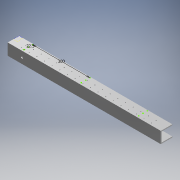
# Autodesk Inventor part: X-portal-front-plate
Saved by Autodesk Inventor 2016 (Build 200138000, 138)
## iProperties
Created: 2015-04-18
Part Number: X-portal-front-plate
Material: Aluminum 6061
Document SubType Name: Modeling
Designer: shu
Density: 2.7 g/cm^3
Appearance: Aluminum - Flat
Mass: 1937.89 g
Surface Area: 2815.57 cm^2
Volume: 717.738 cm^3
Author: shu
Autodesk Inventor part; units mm, degrees
ref_plane "YZ Plane" through (0, 0, 0) normal (1, 0, 0) x (0, 1, 0)
ref_plane "XZ Plane" through (0, 0, 0) normal (0, 1, 0) x (-1, 0, 0)
ref_plane "XY Plane" through (0, 0, 0) normal (0, 0, 1) x (1, 0, 0)
sketch "Sketch1" plane through (0, 0, 0) normal (0, 0, 1) x (1, 0, 0)
  line L0 (0, 0) -> (800, 0)
  line L1 (800, 0) -> (800, -60)
  line L2 (800, -60) -> (0, -60)
  line L3 (0, -60) -> (0, 0)
  dimension "d0" = 800
  dimension "d1" = 60
  constraints: 8 end point, 2 parallel, 1 horizontal, 1 perpendicular
  measures "d0" distance of L1.end L2.end
  measures "d1" distance of L0.end L1.end
extrude "Extrusion1" add sketch "Sketch1" along normal blind 5
sketch "Sketch13" plane through (0, 0, 0) normal (0, 0, -1) x (-1, 0, 0)
  line L0 (0, -60) -> (-800, -60) projected
  line L1 (0, -60) -> (-800, -60)
  line L2 (-800, -60) -> (-800, -55)
  line L3 (-800, -55) -> (0, -55)
  line L4 (0, -55) -> (0, -60)
  point P0 (0, 0)
  dimension "d65" = 800
  dimension "d66" = 5
  constraints: 8 end point, 2 parallel, 1 horizontal, 1 perpendicular
  measures "d65" distance of L2.end L3.end
  measures "d66" distance of L1.end L2.end
extrude "Extrusion12" add sketch "Sketch13" along normal blind 55
sketch "Sketch14" plane through (0, 0, 5) normal (0, 0, 1) x (1, 0, 0)
  line L0 (60, 0) -> (60, -60) construction
  line L1 (0, -60) -> (800, -60) construction
  line L2 (0, -55) -> (0, 0) construction
  point P0 (60, -48)
  point P1 (60, -25)
  dimension "d71" = 60
  constraints: 3 point on line, 2 end point, 1 vertical
  measures "d71" distance from line of L2 point (60, -25)
hole "Hole1" at (60, -48, 5) at (60, -25, 5) direction (0, 0, -1) diameter 4 end through all
pattern_linear "Rectangular Pattern1" count 18 spacing 40 along (1, 0, 0) of "Hole1"
sketch "Sketch15" plane through (0.5, -55, -55) normal (0, 1, 0) x (1, 0, 0)
  line L0 (799.5, 0) -> (-0.5, 0) projected
  line L1 (-0.5, 0) -> (799.5, 0)
  line L2 (799.5, 0) -> (799.5, -5)
  line L3 (799.5, -5) -> (-0.5, -5)
  line L4 (-0.5, -5) -> (-0.5, 0)
  point P0 (-0.5, -55)
  dimension "d91" = 800
  dimension "d92" = 5
  constraints: 8 end point, 2 parallel, 1 horizontal, 1 perpendicular
  measures "d91" distance of L2.end L3.end
  measures "d92" distance of L1.end L2.end
extrude "Extrusion13" add sketch "Sketch15" along normal up to surface (55 mm away)
sketch "Sketch19" plane through (0, -60, 5) normal (0, -1, 0) x (1, 0, 0)
  point P0 (75, -30)
hole "Hole7" at (75, -60, -25) direction (0, 1, 0) diameter 5.3 depth 5 counterbore diameter 10 counterbore depth 3.5
sketch "Sketch20" plane through (0, 0, 5) normal (0, 0, 1) x (1, 0, 0)
  line L0 (0, 0) -> (21.0571, 0) construction
  line L1 (21.0571, 0) -> (21.0571, -30.3151) construction
  line L2 (21.0571, -30.3151) -> (0, -30.3151) construction
  line L3 (0, -30.3151) -> (0, 0) construction
  point P0 (75, -5)
  point P1 (375, -5)
  point P2 (675, -5)
  point P3 (75, -27.5)
  point P4 (375, -27.5)
  point P5 (675, -27.5)
  point P6 (75, -50)
  point P7 (375, -50)
  point P8 (675, -50)
  dimension "d123" = 300
  dimension "d126" = 22.5
  constraints: 8 end point, 2 horizontal, 2 parallel, 1 perpendicular, 1 vertical, 8 other
  measures "d123" distance of point (75, -5) point (375, -5)
  measures "d126" distance of point (75, -5) point (75, -27.5)
sketch "Sketch21" plane through (0, 0, 5) normal (0, 0, 1) x (1, 0, 0)
  point P0 (75, -50)
  point P1 (375, -27.5)
  point P2 (375, -50)
  point P3 (375, -5)
  point P4 (675, -5)
  point P5 (675, -27.5)
  point P6 (675, -50)
  point P7 (75, -5)
  point P8 (75, -27.5)
hole "Hole9" at (75, -50, 5) at (375, -27.5, 5) at (375, -50, 5) at (375, -5, 5) at (675, -5, 5) at (675, -27.5, 5) at (675, -50, 5) at (75, -5, 5) at (75, -27.5, 5) direction (0, 0, -1) diameter 5.5 depth 5
sketch "Sketch22" plane through (0, 0, -55) normal (0, 0, -1) x (-1, 0, 0)
  line L0 (0, 0) -> (-32.4648, 0) construction
  line L1 (-32.4648, 0) -> (-32.4648, -15.4297) construction
  line L2 (-32.4648, -15.4297) -> (0, -15.4297) construction
  line L3 (0, -15.4297) -> (0, 0) construction
  point P0 (-75, -5)
  point P1 (-375, -5)
  point P2 (-675, -5)
  point P3 (-75, -27.5)
  point P4 (-375, -27.5)
  point P5 (-675, -27.5)
  point P6 (-75, -50)
  point P7 (-375, -50)
  point P8 (-675, -50)
  dimension "d138" = 300
  dimension "d141" = 22.5
  constraints: 8 end point, 2 horizontal, 2 parallel, 1 perpendicular, 1 vertical, 8 other
  measures "d138" distance of point (-75, -5) point (-375, -5)
  measures "d141" distance of point (-75, -5) point (-75, -27.5)
hole "Hole11" at (75, -27.5, -55) at (75, -5, -55) at (75, -50, -55) at (375, -50, -55) at (375, -27.5, -55) at (375, -5, -55) at (675, -27.5, -55) at (675, -5, -55) at (675, -50, -55) direction (0, 0, 1) diameter 5 depth 5 tip angle 118
sketch "Sketch23" plane through (0, 0, 0) normal (0, 1, 0) x (1, 0, 0)
  point P0 (200, 52.5)
  point P1 (200, -2.5)
  point P2 (250, -2.5)
  point P3 (300, 52.5)
  point P4 (300, -2.5)
  point P5 (350, 52.5)
  point P6 (350, -2.5)
  point P7 (400, 52.5)
  point P8 (400, -2.5)
  point P9 (450, 52.5)
  point P10 (450, -2.5)
  point P11 (500, 52.5)
  point P12 (500, -2.5)
  point P13 (550, 52.5)
  point P14 (550, -2.5)
  point P15 (600, 52.5)
  point P16 (600, -2.5)
  point P17 (650, 52.5)
  point P18 (650, -2.5)
  point P19 (250, 52.5)
  point P20 (100, 52.5)
  point P21 (100, -2.5)
  point P22 (150, 52.5)
  point P23 (150, -2.5)
hole "Hole12" at (200, 0, -52.5) at (200, 0, 2.5) at (250, 0, 2.5) at (300, 0, -52.5) at (300, 0, 2.5) at (350, 0, -52.5) at (350, 0, 2.5) at (400, 0, -52.5) at (400, 0, 2.5) at (450, 0, -52.5) at (450, 0, 2.5) at (500, 0, -52.5) at (500, 0, 2.5) at (550, 0, -52.5) at (550, 0, 2.5) at (600, 0, -52.5) at (600, 0, 2.5) at (650, 0, -52.5) at (650, 0, 2.5) at (250, 0, -52.5) at (100, 0, -52.5) at (100, 0, 2.5) at (150, 0, -52.5) at (150, 0, 2.5) direction (0, -1, 0) diameter 2.459 depth 15 tip angle 120 thread size "M3x0.5" class "6H" standard "ISO Metric profile"
body "Solid1"
